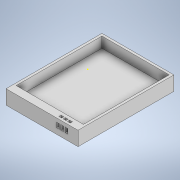
# Autodesk Inventor part: battery-holder
Saved by Autodesk Inventor 2021 (Build 250183000, 183)
## iProperties
Created: 2021-03-31
Part Number: battery-holder
Material: Generic
Document SubType Name: Modeling
Designer: ruby
Density: 1 g/cm^3
Appearance: Default
Author: ruby
Autodesk Inventor part; units mm, degrees
ref_plane "YZ Plane" through (0, 0, 0) normal (1, 0, 0) x (0, 1, 0)
ref_plane "XZ Plane" through (0, 0, 0) normal (0, 1, 0) x (-1, 0, 0)
ref_plane "XY Plane" through (0, 0, 0) normal (0, 0, 1) x (1, 0, 0)
sketch "Sketch2" plane through (0, 0, 0) normal (0, 1, 0) x (-1, 0, 0)
  line L0 (11.0925, -17.7456) -> (-22.3075, -17.7456)
  line L1 (-22.3075, -17.7456) -> (-22.3075, 24.2544)
  line L2 (-22.3075, 24.2544) -> (11.0925, 24.2544)
  line L3 (11.0925, 24.2544) -> (11.0925, -17.7456)
  point P0 (0, 0)
  dimension "d2" = 42
  dimension "d3" = 33.4
  constraints: 8 end point, 2 parallel, 1 horizontal, 1 perpendicular
  measures "d2" distance of L2.end L0.start
  measures "d3" distance of L0.start L0.end
extrude "Extrusion1" add sketch "Sketch2" along normal blind 6
sketch "Sketch3" plane through (0, 6, 0) normal (0, 1, 0) x (1, 0, 0)
  line L0 (-9.9925, 16.6456) -> (21.2075, 16.6456)
  line L1 (21.2075, 16.6456) -> (21.2075, -23.1544)
  line L2 (21.2075, -23.1544) -> (-9.9925, -23.1544)
  line L3 (-9.9925, -23.1544) -> (-9.9925, 16.6456)
  line L4 (22.3075, 17.7456) -> (-11.0925, 17.7456) projected
  line L5 (-11.0925, 17.7456) -> (-11.0925, -24.2544) projected
  line L6 (22.3075, -24.2544) -> (22.3075, 17.7456) projected
  line L7 (-11.0925, -24.2544) -> (22.3075, -24.2544) projected
  point P0 (0, 0)
  dimension "d6" = 1.1
  dimension "d7" = 1.1
  dimension "d8" = 1.1
  dimension "d9" = 1.1
  dimension "d10" = 39.8
  constraints: 8 end point, 2 parallel, 1 horizontal, 1 perpendicular
  measures "d6" distance between parallel lines of L4 L0
  measures "d7" distance between parallel lines of L5 L3
  measures "d8" distance between parallel lines of L6 L1
  measures "d9" distance between parallel lines of L7 L2
  measures "d10" distance of L0.end L1.end
extrude "Extrusion2" cut sketch "Sketch3" against normal blind 4.9 contours L0 L1 L2 L3
sketch "Sketch4" plane through (0, 0, 0) normal (0, -1, 0) x (1, 0, 0)
  line L0 (22.3075, -17.7456) -> (-11.0925, -17.7456) projected
  line L1 (-11.0925, -17.7456) -> (-11.0925, 24.2544) projected
  line L2 (22.3075, -17.7456) -> (-11.0925, -17.7456)
  line L3 (-11.0925, -17.7456) -> (-11.0925, 24.2544)
  line L4 (-11.0925, 24.2544) -> (22.3075, 24.2544)
  line L5 (22.3075, 24.2544) -> (22.3075, -17.7456)
  point P0 (0, 0)
  constraints: 8 end point, 2 parallel, 1 horizontal, 1 perpendicular
extrude "Extrusion3" add sketch "Sketch4" along normal blind 0.6
sketch "Sketch5" plane through (-11.0925, 6, 24.2544) normal (0, 0, 1) x (1, 0, 0)
  line L0 (33.4, -6.6) -> (33.4, 0) projected
  line L1 (33.4, -6.6) -> (0, -6.6)
  line L2 (0, -6.6) -> (0, -2.5)
  line L3 (0, -2.5) -> (33.4, -2.5)
  line L4 (33.4, -2.5) -> (33.4, -6.6)
  point P0 (11.0925, -6)
  point P1 (33.4, -2.5)
  constraints: 8 end point, 2 parallel, 1 horizontal, 1 perpendicular
extrude "Extrusion4" add sketch "Sketch5" along normal blind 3
sketch "Sketch6" plane through (21.2075, 6, 23.1544) normal (0, 0, -1) x (-1, 0, 0)
  line L0 (3.6, -0.9) -> (4.9, -0.9)
  line L1 (4.9, -0.9) -> (4.9, -3.9)
  line L2 (4.9, -3.9) -> (3.6, -3.9)
  line L3 (3.6, -3.9) -> (3.6, -0.9)
  line L4 (0, -4.9) -> (31.2, -4.9) projected
  line L5 (5.6, -0.9) -> (6.9, -0.9)
  line L6 (6.9, -0.9) -> (6.9, -3.9)
  line L7 (6.9, -3.9) -> (5.6, -3.9)
  line L8 (5.6, -3.9) -> (5.6, -0.9)
  line L9 (7.6, -0.9) -> (8.9, -0.9)
  line L10 (8.9, -0.9) -> (8.9, -3.9)
  line L11 (8.9, -3.9) -> (7.6, -3.9)
  line L12 (7.6, -3.9) -> (7.6, -0.9)
  point P0 (21.2075, -6)
  point P1 (0, 0)
  dimension "d17" = 3
  dimension "d18" = 1.3
  dimension "d19" = 3.6
  dimension "d20" = 1
  dimension "d23" = 3
  dimension "d24" = 1.3
  dimension "d25" = 3
  dimension "d26" = 1.3
  dimension "d27" = 1
  dimension "d28" = 1
  dimension "d29" = 0.7
  dimension "d30" = 0.7
  constraints: 24 end point, 6 parallel, 3 horizontal, 3 perpendicular
  measures "d17" distance of L0.end L1.end
  measures "d18" distance of L1.end L2.end
  measures "d19" distance from line of point (0, 0) L3
  measures "d20" distance between parallel lines of L2 L4
  measures "d23" distance of L5.end L6.end
  measures "d24" distance of L6.end L8.start
  measures "d25" distance of L9.end L10.end
  measures "d26" distance of L10.end L12.start
  measures "d27" distance between parallel lines of L4 L7
  measures "d28" distance between parallel lines of L4 L11
  measures "d29" distance between parallel lines of L1 L8
  measures "d30" distance between parallel lines of L6 L12
sketch "Sketch7" plane through (-11.0925, 3.5, 24.2544) normal (0, 1, 0) x (1, 0, 0)
  line L0 (0, 0) -> (33.4, 0) projected
  line L1 (0, 42) -> (0, -3) projected
  line L2 (33.4, 0) -> (0, 0)
  line L3 (0, 0) -> (0, -3)
  line L4 (0, -3) -> (33.4, -3)
  line L5 (33.4, -3) -> (33.4, 0)
  point P0 (11.0925, 24.2544)
  constraints: 8 end point, 2 parallel, 1 horizontal, 1 perpendicular
extrude "Extrusion5" add sketch "Sketch7" along normal blind 2.5
extrude "Extrusion6" cut sketch "Sketch6" against normal through all
sketch "Sketch8" plane through (0, 6, 0) normal (0, 1, 0) x (1, 0, 0)
  point P0 (0, 0)
sketch "Sketch9" plane through (16.3075, 2.1, 23.1544) normal (0, 1, 0) x (1, 0, 0)
  line L0 (1.3, 0) -> (1.3, -4.1) projected
  line L1 (0, 0) -> (0, -4.1) projected
  line L2 (1.3, -2.3) -> (0, -2.3)
  line L3 (0, -2.3) -> (0, -2)
  line L4 (0, -2) -> (1.3, -2)
  line L5 (1.3, -2) -> (1.3, -2.3)
  line L6 (0, 0) -> (1.3, 0) projected
  line L7 (-0.7, -2.3111) -> (-2, -2.3111)
  line L8 (-2, -2.3111) -> (-2, -2.0111)
  line L9 (-2, -2.0111) -> (-0.7, -2.0111)
  line L10 (-0.7, -2.0111) -> (-0.7, -2.3111)
  line L11 (-0.7, 0) -> (-0.7, -4.1) projected
  line L12 (-2, 0) -> (-0.7, 0) projected
  line L13 (-2.7, -2.3) -> (-4, -2.3)
  line L14 (-4, -2) -> (-2.7, -2)
  line L15 (-2.7, -2) -> (-2.7, -2.3)
  line L16 (-4, -2.3) -> (-4, -2)
  line L17 (-4, 0) -> (-2.7, 0) projected
  point P0 (-16.3075, 23.1544)
  point P1 (1.3, -2)
  point P2 (0, -2.3)
  dimension "d33" = 0.3
  dimension "d34" = 2
  dimension "d35" = 0.3
  dimension "d36" = 1.3
  dimension "d37" = 0
  dimension "d38" = 2.0111
  dimension "d39" = 0.3
  dimension "d40" = 1.3
  dimension "d41" = 0
  dimension "d42" = 2
  constraints: 24 end point, 6 parallel, 3 horizontal, 3 perpendicular, 2 point on line
  measures "d33" distance of L4.end L2.start
  measures "d34" distance between parallel lines of L6 L4
  measures "d35" distance of L9.end L7.start
  measures "d36" distance of L9.start L9.end
  measures "d37" distance between parallel lines of L11 L10
  measures "d38" distance between parallel lines of L12 L9
  measures "d39" distance of L14.end L13.start
  measures "d40" distance of L14.start L14.end
  measures "d41" distance from line of L17.end L15
  measures "d42" distance between parallel lines of L17 L14
extrude "Extrusion7" add sketch "Sketch9" along normal up to surface (3.9 mm away) contours L0 L2 L1 L4 | L7 L8 L9 L10 | L13 L16 L14 L15
sketch "Sketch10" plane through (0, 6, 0) normal (0, 1, 0) x (1, 0, 0)
  line L0 (17.6075, -25.6544) -> (16.3075, -25.6544)
  line L1 (16.3075, -25.6544) -> (16.3075, -24.6544)
  line L2 (16.3075, -24.6544) -> (17.6075, -24.6544)
  line L3 (17.6075, -24.6544) -> (17.6075, -25.6544)
  line L4 (21.2075, -23.1544) -> (-9.9925, -23.1544) projected
  line L5 (13.6075, -25.6544) -> (12.3075, -25.6544)
  line L6 (12.3075, -25.6544) -> (12.3075, -24.6544)
  line L7 (12.3075, -24.6544) -> (13.6075, -24.6544)
  line L8 (13.6075, -24.6544) -> (13.6075, -25.6544)
  line L9 (15.6075, -25.6544) -> (14.3075, -25.6544)
  line L10 (14.3075, -25.6544) -> (14.3075, -24.6544)
  line L11 (14.3075, -24.6544) -> (15.6075, -24.6544)
  line L12 (15.6075, -24.6544) -> (15.6075, -25.6544)
  line L13 (13.6075, -25.4544) -> (13.6075, -27.2544) projected
  point P0 (0, 0)
  point P1 (17.6075, -23.1544)
  point P2 (15.6075, -27.2544)
  dimension "d45" = 1.3
  dimension "d46" = 1
  dimension "d47" = 0
  dimension "d48" = 1.5
  dimension "d49" = 1.3
  dimension "d50" = 1
  dimension "d51" = 1.3
  dimension "d52" = 1
  dimension "d53" = 1.5
  dimension "d54" = 1.5
  dimension "d55" = 0
  dimension "d56" = 0
  constraints: 24 end point, 6 parallel, 3 horizontal, 3 perpendicular
  measures "d45" distance of L1.end L2.end
  measures "d46" distance of L2.end L0.start
  measures "d47" distance from line of point (17.607, -23.154) L3
  measures "d48" distance between parallel lines of L4 L2
  measures "d49" distance of L6.end L8.start
  measures "d50" distance of L8.start L5.start
  measures "d51" distance of L10.end L12.start
  measures "d52" distance of L12.start L9.start
  measures "d53" distance between parallel lines of L4 L11
  measures "d54" distance between parallel lines of L4 L7
  measures "d55" distance between parallel lines of L13 L8
  measures "d56" distance from line of point (15.607, -27.254) L12
extrude "Extrusion8" cut sketch "Sketch10" against normal blind 1.5
sketch "Sketch11" plane through (-11.0925, 6, 27.2544) normal (0, 0, 1) x (1, 0, 0)
  line L0 (28.7, 0) -> (28.7, -0.9) projected
  line L1 (27.4, -3.9) -> (27.4, -0.9) projected
  line L2 (28.7, -0.9) -> (27.4, -0.9)
  line L3 (27.4, -0.9) -> (27.4, -1.7)
  line L4 (27.4, -1.7) -> (28.7, -1.7)
  line L5 (28.7, -1.7) -> (28.7, -0.9)
  line L6 (26.7, 0) -> (26.7, -0.9) projected
  line L7 (25.4, -3.9) -> (25.4, -1.5) projected
  line L8 (26.7, -0.9) -> (25.4, -0.9)
  line L9 (25.4, -0.9) -> (25.4, -1.7)
  line L10 (25.4, -1.7) -> (26.7, -1.7)
  line L11 (26.7, -1.7) -> (26.7, -0.9)
  line L12 (24.7, -0.9) -> (24.7, -3.9) projected
  line L13 (23.4, -3.9) -> (23.4, -0.9) projected
  line L14 (24.7, -0.9) -> (23.4, -0.9)
  line L15 (23.4, -0.9) -> (23.4, -1.7)
  line L16 (23.4, -1.7) -> (24.7, -1.7)
  line L17 (24.7, -1.7) -> (24.7, -0.9)
  point P0 (11.0925, -6)
  point P1 (24.7, -1.7)
  dimension "d59" = 0.8
  constraints: 24 end point, 6 parallel, 5 point on line, 3 horizontal, 3 perpendicular
  measures "d59" distance of L4.end L0.end
extrude "Extrusion9" add sketch "Sketch11" against normal up to surface (1.6 mm away)
sketch "Sketch12" plane through (0, 6, 0) normal (0, 1, 0) x (1, 0, 0)
  line L0 (-11.0925, -27.2544) -> (22.3075, -27.2544) projected
  line L1 (-11.0925, 17.7456) -> (-11.0925, -27.2544) projected
  line L2 (22.3075, -27.2544) -> (-11.0925, -27.2544)
  line L3 (-11.0925, -27.2544) -> (-11.0925, -26.7544)
  line L4 (-11.0925, -26.7544) -> (22.3075, -26.7544)
  line L5 (22.3075, -26.7544) -> (22.3075, -27.2544)
  line L6 (17.6075, -25.6544) -> (16.3075, -25.6544) projected
  point P0 (0, 0)
  dimension "d62" = 1.1
  constraints: 8 end point, 2 parallel, 1 horizontal, 1 perpendicular, 1 point on line
  measures "d62" distance between parallel lines of L6 L4
extrude "Extrusion10" cut sketch "Sketch12" against normal through all
body "Solid1"
